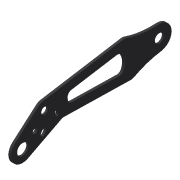
# Autodesk Inventor part: UPPER_LEG_OUTER_FRAME
Saved by Autodesk Inventor 2019.4 (Build 234330000, 330)
## iProperties
Created: 2019-11-12
Part Number: UPPER_LEG_OUTER_FRAME
Material: 一般
Document SubType Name: Modeling
Designer: y6tada
Density: 1 g/cm^3
Appearance: Black 80
Mass: 5.99749 g
Surface Area: 71.6947 cm^2
Volume: 5.99749 cm^3
Author: y6tada
Autodesk Inventor part; units mm, degrees
ref_plane "YZ Plane" through (0, 0, 0) normal (1, 0, 0) x (0, 1, 0)
ref_plane "XZ Plane" through (0, 0, 0) normal (0, 1, 0) x (-1, 0, 0)
ref_plane "XY Plane" through (0, 0, 0) normal (0, 0, 1) x (1, 0, 0)
sketch "スケッチ1" plane through (0, 0, 0) normal (1, 0, 0) x (0, 1, 0)
  line L0 (0, 0) -> (0, 125) construction
  arc A0 (10.4476, 126.4665) -> (-10.542, 124.5901) centre (0, 125) ccw
  arc A1 (9.5221, 125.7296) -> (-7.8176, 119.5148) centre (0, 125) ccw construction
  line L1 (9.5221, 125.7296) -> (19.0442, 1.4592) construction
  line L2 (-7.8176, 119.5148) -> (-1.1797, 110.0544) construction
  arc A2 (-0.7923, 105.8489) -> (-1.1797, 110.0544) centre (-4.6587, 107.6133) ccw construction
  circle A3 centre (-4.6587, 107.6133) radius 4
  arc A4 (-4.5464, 108.0035) -> (-4.7566, 107.2192) centre (5.9664, 104.7663) ccw construction
  circle A5 centre (5.9664, 104.7663) radius 1.6 construction
  arc A6 (17.3156, 27.8342) -> (10.9958, -0.3023) centre (85.9675, -2.3638) ccw
  arc A7 (-10.9929, -0.3964) -> (10.9958, -0.3023) centre (0, 0) ccw
  arc A8 (-10.9929, -0.3964) -> (-17.5957, 27.7797) centre (-85.9441, -3.099) ccw
  line L3 (-15.1422, 75.5391) -> (-18.1148, 30.6464)
  line L4 (5.9664, 104.7663) -> (-4.6587, 107.6133) construction
  arc A9 (-18.742, 3.6807) -> (19.0442, 1.4592) centre (0, 0) ccw construction
  arc A10 (17.3156, 27.8342) -> (17.8229, 30.3321) centre (11.8235, 30.25) ccw
  arc A11 (-18.1148, 30.6464) -> (-17.5957, 27.7797) centre (-12.1279, 30.25) ccw
  line L5 (10.9958, -0.3023) -> (0, 0) construction
  line L6 (0, 0) -> (-10.9929, -0.3964) construction
  line L7 (9.4327, 35.2736) -> (6.8063, 69.5498)
  line L8 (-7.9258, 63.4396) -> (-9.7871, 35.3299)
  arc A12 (-6.8998, 31.221) -> (6.4814, 31.1048) centre (0, 55.25) ccw
  arc A13 (6.4814, 31.1048) -> (9.4327, 35.2736) centre (5.4444, 34.968) ccw
  arc A14 (-9.7871, 35.3299) -> (-6.8998, 31.221) centre (-5.7959, 35.0656) ccw
  arc A15 (-5.4818, 66.8639) -> (-7.9258, 63.4396) centre (-3.9346, 63.1753) ccw
  line L9 (-0.7923, 105.8489) -> (-13.5138, 77.9726) construction
  line L10 (-14.1444, 75.4731) -> (-19.3486, -3.1223) construction
  arc A16 (-13.5138, 77.9726) -> (-14.1444, 75.4731) centre (-7, 75) ccw construction
  arc A17 (-14.9577, 76.8059) -> (-15.1422, 75.5391) centre (-7, 75) ccw
  circle A18 centre (-4.6587, 107.6133) radius 6 construction
  arc A19 (6.9396, 102.6901) -> (7.8473, 106.0778) centre (-4.6587, 107.6133) ccw
  arc A20 (3.994, 103.9405) -> (4.6712, 106.4678) centre (-4.6587, 107.6133) ccw
  arc A21 (7.8473, 106.0778) -> (4.6712, 106.4678) centre (6.2593, 106.2728) ccw
  arc A22 (3.994, 103.9405) -> (6.9396, 102.6901) centre (5.4668, 103.3153) ccw
  line L11 (6.2593, 106.2728) -> (-4.6587, 107.6133) construction
  line L12 (-4.6587, 107.6133) -> (5.4668, 103.3153) construction
  line L13 (11.8235, 30.25) -> (-12.1279, 30.25) construction
  arc A23 (6.8063, 69.5498) -> (1.7829, 71.5275) centre (3.8151, 69.3206) ccw
  arc A24 (-5.4818, 66.8639) -> (1.7829, 71.5275) centre (-15.1521, 89.9179) ccw
  arc A25 (17.8229, 30.3321) -> (10.4476, 126.4665) centre (-749.1865, 19.8382) ccw
  line L14 (12.0148, 125.9206) -> (21.5369, 1.6502) construction
  line L15 (11.4747, 113.335) -> (17.1037, 39.8734) construction
  arc A26 (-14.9577, 76.8059) -> (-10.542, 124.5901) centre (-194.0689, 117.4533) ccw
  line L16 (0, 125) -> (-4.6587, 107.6133) construction
  circle A27 centre (-7, 75) radius 8 construction
  line L17 (3.8151, 69.3206) -> (-3.9346, 63.1753) construction
  line L18 (-7, 75) -> (-0.0598, 66.2479) construction
  point P0 (-14.406, 86.6566)
  point P1 (17.9231, 29.1792)
  point P2 (-14.4228, 86.4034)
  point P3 (-9.9857, 32.3309)
  point P4 (9.6685, 32.1953)
  point P5 (7.074, 66.0557)
  dimension "d2" = 125
  dimension "d10" = 19.1
  dimension "d13" = 8
  dimension "d14" = 0.25
  dimension "d20" = 3.2
  dimension "d25" = 11
  dimension "d75" = 19.1
  dimension "d79" = 1
  dimension "d86" = 6
  dimension "d87" = 75
  dimension "d95" = 8
  dimension "d96" = 4
  dimension "d109" = 1
  dimension "d111" = 75
  dimension "d116" = 12
  dimension "d117" = 11
  dimension "d118" = 16
  dimension "d119" = 30.25
  dimension "d120" = 25
  dimension "d124" = 3
  dimension "d128" = 25
  dimension "d130" = 2.5
  dimension "d131" = 8
  dimension "d132" = 18
  dimension "d133" = 15
  dimension "d134" = 7
  dimension "d135" = 16
  dimension "d136" = 7.16
  constraints: 52 point on circle, 40 end point, 38 tangent, 28 centre point, 13 coincident, 6 point on line, 4 equal radius, 4 parallel, 3 concentric, 2 perpendicular, 1 horizontal, 1 midpoint, 1 symmetric about line, 1 vertical
  measures "d2" distance of L0.end L0.start
  measures "d10" diameter of A1
  measures "d13" diameter of A3
  measures "d14" radial gap between concentric circles of A3 A2
  measures "d20" diameter of A5
  measures "d25" radius of A7
  measures "d75" radius of A9
  measures "d79" radial gap between concentric circles of A0 A1
  measures "d86" radius of A10
  measures "d87" radius of A6
  measures "d95" distance between parallel lines of L3 L8
  measures "d96" radius of A13
  measures "d109" distance between parallel lines of L3 L10
  measures "d111" vertical distance of L0.start A16.centre
  measures "d116" diameter of A18
  measures "d117" distance of L4.start L4.end
  measures "d118" angle of L12 L11
  measures "d119" distance from line of L0.start L13
  measures "d120" radius of A12
  measures "d124" radius of A23
  measures "d128" radius of A24
  measures "d130" distance between parallel lines of L1 L14
  measures "d131" distance between parallel lines of L7 L15
  measures "d132" distance of L16.start L11.end
  measures "d133" angle of L0 L16
  measures "d134" distance from line of L0 point (-7, 75)
  measures "d135" diameter of A27
  measures "d136" radius of A16
extrude "押し出し1" add sketch "スケッチ1" along normal blind 2
hole "穴1" at (0, 0, 0) direction (1, 0, 0) diameter 8 end through all counterbore diameter 9.3 counterbore depth 0.65
hole "穴2" at (0, -7, 75) direction (1, 0, 0) diameter 6 end through all counterbore diameter 7.3 counterbore depth 0.65
hole "穴3" at (0, 0, 125) direction (1, 0, 0) diameter 10 end through all counterbore diameter 11.3 counterbore depth 0.65
